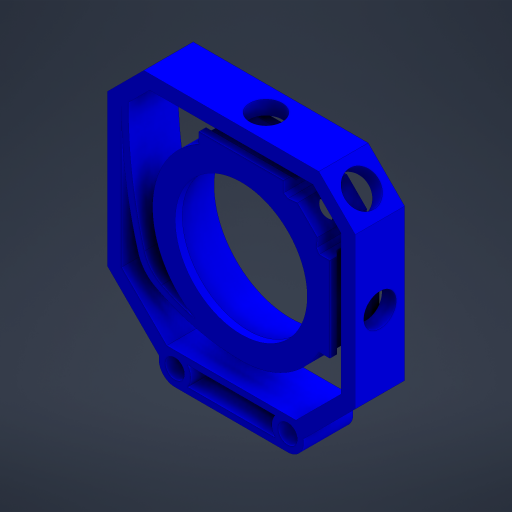
# Autodesk Inventor part: One Inch Lense Holder (V5)
Saved by Autodesk Inventor 2023.4 (Build 274418000, 418)
## iProperties
Created: 2022-07-25
Part Number: One Inch Lense Holder (V5)
Material: Generic
Document SubType Name: Modeling
Designer: xSibe
Density: 1 g/cm^3
Appearance: Plastic Blue
Author: xSibe
Autodesk Inventor part; units mm, degrees
ref_plane "YZ Plane" through (0, 0, 0) normal (1, 0, 0) x (0, 1, 0)
ref_plane "XZ Plane" through (0, 0, 0) normal (0, 1, 0) x (-1, 0, 0)
sketch "Sketch1" plane through (0, 0, 0) normal (0, 0, 1) x (1, 0, 0)
  circle A0 centre (139.6, 3.85) radius 2.8125
  circle A1 centre (159.6, 3.85) radius 2.8125
  line L0 (159.6, 1.0375) -> (139.6, 1.0375)
  line L1 (149.6, 24.9) -> (151.367767, 26.667767)
  line L2 (149.6, 24.9) -> (152.1, 24.9) construction
  circle A2 centre (151.367767, 26.667767) radius 13.575
  circle A3 centre (151.367767, 26.667767) radius 11.075
  circle A4 centre (151.367767, 26.667767) radius 15.7
  line L3 (151.367767, 26.667767) -> (151.367767, 42.367767)
  line L4 (151.367767, 42.367767) -> (151.367767, 41.367767)
  line L5 (143.867767, 40.367767) -> (158.867767, 40.367767)
  line L6 (158.867767, 40.367767) -> (158.867767, 42.367767)
  line L7 (158.867767, 42.367767) -> (143.867767, 42.367767)
  line L8 (143.867767, 42.367767) -> (143.867767, 40.367767)
  line L9 (143.867767, 40.367767) -> (158.867767, 42.367767) construction
  line L10 (158.867767, 40.367767) -> (143.867767, 42.367767) construction
  line L11 (151.367767, 26.667767) -> (162.469343, 37.769343)
  line L12 (162.469343, 37.769343) -> (162.027402, 37.327402)
  line L13 (164.855829, 36.620295) -> (161.320295, 40.155829)
  line L14 (161.320295, 40.155829) -> (159.198975, 38.034508)
  line L15 (159.198975, 38.034508) -> (162.734508, 34.498975)
  line L16 (162.734508, 34.498975) -> (164.855829, 36.620295)
  line L17 (164.855829, 36.620295) -> (159.198975, 38.034508) construction
  line L18 (161.320295, 40.155829) -> (162.734508, 34.498975) construction
  line L19 (164.855829, 36.620295) -> (169.855829, 36.620295) construction
  line L20 (165.067767, 19.167767) -> (165.067767, 34.167767)
  line L21 (165.067767, 34.167767) -> (167.067767, 34.167767)
  line L22 (167.067767, 34.167767) -> (167.067767, 19.167767)
  line L23 (167.067767, 19.167767) -> (165.067767, 19.167767)
  line L24 (151.367767, 42.367767) -> (151.367767, 44.367767)
  line L25 (167.067767, 26.667767) -> (169.067767, 26.667767)
  line L26 (139.382233, 5.432233) -> (159.817767, 5.432233)
  line L27 (169.067767, 14.682233) -> (169.067767, 39.367767)
  line L28 (164.067767, 44.367767) -> (135.132233, 44.367767)
  line L29 (130.132233, 39.367767) -> (130.132233, 14.682233)
  line L30 (130.132233, 5.432233) -> (169.067767, 44.367767) construction
  line L31 (169.067767, 5.432233) -> (130.132233, 44.367767) construction
  line L32 (139.382233, 5.432233) -> (130.132233, 14.682233)
  line L33 (159.817767, 5.432233) -> (169.067767, 14.682233)
  line L34 (164.067767, 44.367767) -> (169.067767, 39.367767)
  line L35 (135.132233, 44.367767) -> (130.132233, 39.367767)
  line L36 (134.096699, 46.867767) -> (127.632233, 40.403301)
  line L37 (127.632233, 40.403301) -> (127.632233, 13.646699)
  line L38 (127.632233, 13.646699) -> (138.346699, 2.932233)
  line L39 (138.346699, 2.932233) -> (160.853301, 2.932233)
  line L40 (160.853301, 2.932233) -> (171.567767, 13.646699)
  line L41 (171.567767, 13.646699) -> (171.567767, 40.403301)
  line L42 (171.567767, 40.403301) -> (165.103301, 46.867767)
  line L43 (165.103301, 46.867767) -> (134.096699, 46.867767)
  circle A5 centre (139.6, 3.85) radius 1.705
  circle A6 centre (159.6, 3.85) radius 1.705
  line L44 (151.367767, 10.967767) -> (133.867767, 10.967767)
  arc A7 (133.867767, 15.967767) -> (151.367767, 10.967767) centre (151.367767, 44.092767) ccw
  line L45 (133.867767, 10.967767) -> (133.867767, 15.967767)
  arc A8 (130.132233, 39.367767) -> (133.867767, 15.967767) centre (205.290728, 39.367767) ccw
  arc A9 (131.392987, 40.628521) -> (134.914424, 16.792526) centre (205.290728, 39.367767) ccw
  arc A10 (134.914424, 16.792526) -> (143.135448, 13.299187) centre (151.367767, 44.092767) ccw
  arc A11 (133.129032, 18.356128) -> (136.173995, 14.65784) centre (138.95926, 20.053742) ccw
  line L46 (133.867767, 15.967767) -> (133.129032, 18.356128)
  line L47 (134.914424, 16.792526) -> (134.191173, 19.185622)
  arc A12 (134.191173, 19.185622) -> (137.244434, 15.517479) centre (139.851544, 20.792361) ccw
  line L48 (132.55, 7.7) -> (132.55, 42.1)
  line L49 (166.65, 7.7) -> (166.65, 42.1)
  line L50 (132.55, 24.9) -> (166.65, 24.9)
  circle A13 centre (139.6, 3.85) radius 1.5625
  circle A14 centre (159.6, 3.85) radius 1.5625
  line L51 (139.6, 5.555) -> (159.6, 5.555)
  line L52 (139.6, 2.145) -> (159.6, 2.145)
  line L53 (138.151966, 6.6625) -> (161.048034, 6.6625)
  point P0 (56.607839, -34.156627)
  point P1 (156.941455, 2.932233)
  point P2 (142.258545, 2.932233)
  point P3 (138.414176, 6.40029)
  point P4 (160.785824, 6.40029)
  point P5 (143.867767, 40.460519)
  point P6 (165.160519, 19.167767)
  point P7 (165.160519, 34.167767)
  point P8 (164.095461, 35.859927)
  point P9 (160.559927, 39.395461)
  point P10 (158.867767, 40.460519)
  point P11 (162.351875, 4.430808)
  point P12 (136.848125, 4.430808)
  point P13 (-7.831162, 14.243977)
  point P14 (157.27477, 5.432233)
  point P15 (141.92523, 5.432233)
  point P16 (133.188717, 18.163163)
  point P17 (134.248753, 18.995103)
  point P18 (167.067767, 26.667767)
  point P19 (141.836768, 5.555)
  point P20 (157.363232, 5.555)
  point P21 (157.363232, 2.145)
  point P22 (141.836768, 2.145)
  dimension "d2" = 2.5
  dimension "d3" = 45
  dimension "d4" = 27.15
  dimension "d5" = 2.5
  dimension "d6" = 2.125
  dimension "d7" = 1
  dimension "d8" = 15
  dimension "d9" = 2
  dimension "d10" = 0.625
  dimension "d11" = 5
  dimension "d12" = 135
  dimension "d13" = 3
  dimension "d14" = 2
  dimension "d15" = 2
  dimension "d16" = 38.93553
  dimension "d17" = 38.93553
  dimension "d18" = 9.25
  dimension "d19" = 9.25
  dimension "d20" = 9.25
  dimension "d21" = 9.25
  dimension "d22" = 5
  dimension "d23" = 5
  dimension "d24" = 5
  dimension "d25" = 5
  dimension "d26" = 2.5
  dimension "d48" = 17.5
  dimension "d49" = 5
  dimension "d50" = 1.25
  dimension "d51" = 2.5
  dimension "d52" = 2.5
  dimension "d56" = 0.1425
  dimension "d57" = 0.1425
  dimension "d58" = 1.25
  dimension "d60" = 1.25
  constraints: 104 end point, 24 point on circle, 15 point on line, 11 centre point, 11 tangent, 10 horizontal, 10 midpoint, 8 parallel, 6 perpendicular, 4 symmetric about line, 3 coincident, 2 equal length, 2 vertical, 14 other
  measures "d2" distance of L1.start L1.end
  measures "d3" angle of L2 L1
  measures "d4" diameter of A2
  measures "d5" radial gap between concentric circles of A2 A3
  measures "d6" radial gap between concentric circles of A2 A4
  measures "d7" distance of L3.end L4.end
  measures "d8" distance of L7.end L6.end
  measures "d9" distance of L6.end L5.end
  measures "d10" distance of L11.end L12.end
  measures "d11" distance of L13.start L13.end
  measures "d12" angle of L19 L13
  measures "d13" distance of L14.end L13.end
  measures "d14" distance of L3.end L24.end
  measures "d15" distance of L25.start L25.end
  measures "d16" distance of L30.end L31.end
  measures "d17" distance of L31.end L30.start
  measures "d18" distance of L26.start L30.start
  measures "d19" distance of L29.end L30.start
  measures "d20" distance of L26.end L31.start
  measures "d21" distance of L27.start L31.start
  measures "d22" distance of L28.start L30.end
  measures "d23" distance of L27.end L30.end
  measures "d24" distance of L28.end L31.end
  measures "d25" distance of L29.start L31.end
  measures "d26" distance between parallel lines of L28 L43
  measures "d48" distance of L44.start L44.end
  measures "d49" distance of L44.end L45.end
  measures "d50" radial gap between concentric circles of A8 A9
  measures "d51" distance of L45.end L46.end
  measures "d52" distance of L47.start L47.end
  measures "d56" radial gap between concentric circles of A13 A5
  measures "d57" radial gap between concentric circles of A14 A6
sketch "Sketch1 outline for Extrusion1" plane through (0, 0, 0) normal (0, 0, 1) x (1, 0, 0)
  line L0 (157.363232, 2.145) -> (141.836768, 2.145)
  arc A0 (141.836768, 2.145) -> (141.836768, 5.555) centre (139.6, 3.85) ccw
  line L1 (141.836768, 5.555) -> (157.363232, 5.555)
  arc A1 (157.363232, 5.555) -> (157.363232, 2.145) centre (159.6, 3.85) ccw
  line L2 (139.6, 1.0375) -> (159.6, 1.0375)
  arc A2 (159.6, 1.0375) -> (162.351875, 4.430808) centre (159.6, 3.85) ccw
  line L3 (162.351875, 4.430808) -> (171.567767, 13.646699)
  line L4 (171.567767, 13.646699) -> (171.567767, 40.403301)
  line L5 (171.567767, 40.403301) -> (165.103301, 46.867767)
  line L6 (165.103301, 46.867767) -> (134.096699, 46.867767)
  line L7 (134.096699, 46.867767) -> (127.632233, 40.403301)
  line L8 (127.632233, 40.403301) -> (127.632233, 13.646699)
  line L9 (127.632233, 13.646699) -> (136.848125, 4.430808)
  arc A3 (136.848125, 4.430808) -> (139.6, 1.0375) centre (139.6, 3.85) ccw
  line L10 (158.867767, 40.460519) -> (158.867767, 42.367767)
  line L11 (158.867767, 42.367767) -> (143.867767, 42.367767)
  line L12 (143.867767, 42.367767) -> (143.867767, 40.460519)
  arc A4 (143.867767, 40.460519) -> (143.135448, 13.299187) centre (151.367767, 26.667767) ccw
  arc A5 (143.135448, 13.299187) -> (137.244434, 15.517479) centre (151.367767, 44.092767) cw
  arc A6 (137.244434, 15.517479) -> (134.191173, 19.185622) centre (139.851544, 20.792361) cw
  arc A7 (134.191173, 19.185622) -> (131.392987, 40.628521) centre (205.290728, 39.367767) cw
  line L13 (131.392987, 40.628521) -> (135.132233, 44.367767)
  line L14 (135.132233, 44.367767) -> (164.067767, 44.367767)
  line L15 (164.067767, 44.367767) -> (169.067767, 39.367767)
  line L16 (169.067767, 39.367767) -> (169.067767, 14.682233)
  line L17 (169.067767, 14.682233) -> (161.048034, 6.6625)
  line L18 (161.048034, 6.6625) -> (138.151966, 6.6625)
  line L19 (138.151966, 6.6625) -> (130.132233, 14.682233)
  line L20 (130.132233, 14.682233) -> (130.132233, 39.367767)
  arc A8 (130.132233, 39.367767) -> (133.129032, 18.356128) centre (205.290728, 39.367767) ccw
  arc A9 (133.129032, 18.356128) -> (136.173995, 14.65784) centre (138.95926, 20.053742) ccw
  arc A10 (136.173995, 14.65784) -> (151.367767, 10.967767) centre (151.367767, 44.092767) ccw
  arc A11 (151.367767, 10.967767) -> (165.160519, 19.167767) centre (151.367767, 26.667767) ccw
  line L21 (165.160519, 19.167767) -> (167.067767, 19.167767)
  line L22 (167.067767, 19.167767) -> (167.067767, 34.167767)
  line L23 (167.067767, 34.167767) -> (165.160519, 34.167767)
  arc A12 (165.160519, 34.167767) -> (164.095461, 35.859927) centre (151.367767, 26.667767) ccw
  line L24 (164.095461, 35.859927) -> (164.855829, 36.620295)
  line L25 (164.855829, 36.620295) -> (161.320295, 40.155829)
  line L26 (161.320295, 40.155829) -> (160.559927, 39.395461)
  arc A13 (160.559927, 39.395461) -> (158.867767, 40.460519) centre (151.367767, 26.667767) ccw
  circle A14 centre (151.367767, 26.667767) radius 13.575
  circle A15 centre (139.6, 3.85) radius 1.705
  circle A16 centre (159.6, 3.85) radius 1.705
extrude "Extrusion1" add sketch "Sketch1 outline for Extrusion1" along normal mid plane 8.75
sketch "Sketch2" plane through (0, 0, 0) normal (0, 0, 1) x (1, 0, 0)
  circle A0 centre (151.367767, 26.667767) radius 13.575
  circle A1 centre (151.367767, 26.667767) radius 11.7
  point P0 (0, 0)
  dimension "d30" = 1.875
  constraints: 1 centre point
  measures "d30" radial gap between concentric circles of A0 A1
sketch "Sketch2 outline for Extrusion2" plane through (0, 0, 0) normal (0, 0, 1) x (1, 0, 0)
  circle A0 centre (151.367767, 26.667767) radius 13.575
  circle A1 centre (151.367767, 26.667767) radius 11.7
extrude "Extrusion2" add sketch "Sketch2 outline for Extrusion2" against normal blind 1.25 from surface at 4.375
sketch "Sketch3" plane through (171.567767, 13.646699, -4.375) normal (1, 0, 0) x (0, 0, -1)
  line L0 (0, 5.521068) -> (-8.75, 5.521068)
  line L1 (0, 20.521068) -> (0, 5.521068)
  line L2 (0, 20.521068) -> (-8.75, 20.521068)
  line L3 (-8.75, 5.521068) -> (-8.75, 20.521068)
  line L4 (-4.375, 20.521068) -> (-4.375, 5.521068)
  circle A0 centre (-4.375, 13.021068) radius 2.875
  point P0 (-4.375, -13.646699)
  dimension "d33" = 5.75
  constraints: 3 midpoint, 2 end point, 1 centre point
  measures "d33" diameter of A0
sketch "Sketch3 outline for Extrusion3" plane through (171.567767, 13.646699, -4.375) normal (1, 0, 0) x (0, 0, -1)
  circle A0 centre (-4.375, 13.021068) radius 2.875
extrude "Extrusion3" cut sketch "Sketch3 outline for Extrusion3" against normal up to surface (2.5 mm away)
sketch "Sketch4" plane through (165.160519, 34.167767, -4.375) normal (0, 1, 0) x (1, 0, 0)
  line L0 (1.907248, 0) -> (1.907248, -8.75)
  line L1 (0, 0) -> (1.907248, 0)
  line L2 (0, 0) -> (0, -8.75)
  line L3 (1.907248, -8.75) -> (0, -8.75)
  line L4 (1.907248, -8.75) -> (0, -8.75)
  line L5 (0, -8.75) -> (0, -7.5)
  line L6 (0, -7.5) -> (1.907248, -7.5)
  line L7 (1.907248, -7.5) -> (1.907248, -8.75)
  line L8 (1.907248, -7.5) -> (0, -5.592752)
  line L9 (1.907248, -7.5) -> (4.604505, -7.5) construction
  line L10 (0, -4.375) -> (1.907248, -4.375)
  line L11 (1.907248, -1.25) -> (0, -3.157248)
  line L12 (0.953624, -8.75) -> (0.953624, 0)
  point P0 (-165.160519, -4.375)
  point P1 (1.907248, -1.25)
  point P2 (0, -3.157248)
  point P3 (1.907248, -7.5)
  point P4 (0.953624, -2.203624)
  point P5 (0.953624, -6.546376)
  dimension "d36" = 1.25
  dimension "d37" = 135
  constraints: 18 end point, 4 midpoint, 2 horizontal, 2 parallel, 2 point on line, 2 symmetric about line, 1 equal length, 1 perpendicular
  measures "d36" distance of L4.end L5.end
  measures "d37" angle of L9 L8
sketch "Sketch4 outline for Extrusion4" plane through (165.160519, 34.167767, -4.375) normal (0, 1, 0) x (1, 0, 0)
  line L0 (0.953624, -2.203624) -> (0.953624, -6.546376)
  line L1 (1.907248, -1.25) -> (0.953624, -2.203624)
  line L2 (1.907248, -7.5) -> (1.907248, -1.25)
  line L3 (0.953624, -6.546376) -> (1.907248, -7.5)
extrude "Extrusion4" cut sketch "Sketch4 outline for Extrusion4" against normal up to surface (15 mm away)
ref_plane "Work Plane1" through (167.067767, 42.367767, 4.375) normal (0.7071068, -0.7071068, 0) x (0, 0, -1)
mirror "Mirror1" about plane through (167.067767, 42.367767, 4.375) normal (0.7071068, -0.7071068, 0) of "Extrusion3", "Extrusion4"
sketch "Sketch5" plane through (171.567767, 40.403301, 4.375) normal (0.7071068, 0.7071068, 0) x (0.7071068, -0.7071068, 0)
  line L0 (0, 8.75) -> (0, 0)
  line L1 (-9.142136, 8.75) -> (0, 8.75)
  line L2 (-9.142136, 8.75) -> (-9.142136, 0)
  line L3 (0, 0) -> (-9.142136, 0)
  line L4 (-2.071068, 8.75) -> (-2.071068, 0)
  line L5 (-7.071068, 8.75) -> (-2.071068, 8.75)
  line L6 (-7.071068, 8.75) -> (-7.071068, 0)
  line L7 (-2.071068, 0) -> (-7.071068, 0)
  circle A0 centre (-4.571068, 4.375) radius 1.875
  line L8 (-7.071068, 4.375) -> (-2.071068, 4.375)
  circle A1 centre (-4.571068, 4.375) radius 3
  dimension "d40" = 3.75
  dimension "d41" = 6
  constraints: 3 midpoint, 2 centre point, 2 end point, 1 coincident
  measures "d40" diameter of A0
  measures "d41" diameter of A1
sketch "Sketch5 outline for Extrusion5" plane through (171.567767, 40.403301, 4.375) normal (0.7071068, 0.7071068, 0) x (0.7071068, -0.7071068, 0)
  circle A0 centre (-4.571068, 4.375) radius 3
extrude "Extrusion5" cut sketch "Sketch5 outline for Extrusion5" against normal up to surface (2.5 mm away)
sketch "Sketch5 outline for Extrusion6" plane through (171.567767, 40.403301, 4.375) normal (0.7071068, 0.7071068, 0) x (0.7071068, -0.7071068, 0)
  circle A0 centre (-4.571068, 4.375) radius 1.875
extrude "Extrusion6" cut sketch "Sketch5 outline for Extrusion6" against normal up to next from surface at -7.421046
chamfer "Chamfer1" distance 1.075 angle 45 2 edges at (164.0955, 35.8599, 0) (160.5599, 39.3955, 0)
equation "\"d19\" = d18"
equation "\"d20\" = d18"
equation "\"d21\" = d20"
equation "\"d23\" = d22"
equation "\"d24\" = d22"
equation "\"d25\" = d24"
body "Solid1"
